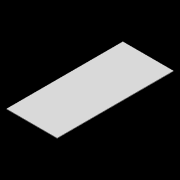
# Autodesk Inventor part: AirPlate
Saved by Autodesk Inventor 2022 (Build 260153000, 153)
## iProperties
Created: 2021-10-09
Part Number: AirPlate
Material: Generic
Document SubType Name: Modeling
Designer: timmy
Density: 1 g/cm^3
Appearance: Default
Author: timmy
Autodesk Inventor part; units mm, degrees
ref_plane "YZ Plane" through (0, 0, 0) normal (1, 0, 0) x (0, 1, 0)
ref_plane "XZ Plane" through (0, 0, 0) normal (0, 1, 0) x (-1, 0, 0)
ref_plane "XY Plane" through (0, 0, 0) normal (0, 0, 1) x (1, 0, 0)
sketch "Sketch1" plane through (0, 0, 0) normal (0, 1, 0) x (-1, 0, 0)
  line L0 (0, 0) -> (188.2648, 0)
  line L1 (188.2648, 0) -> (188.2648, -431.8)
  line L2 (188.2648, -431.8) -> (0, -431.8)
  line L3 (0, -431.8) -> (0, 0)
  dimension "d0" = 188.2648
  dimension "d1" = 431.8
  constraints: 8 end point, 2 parallel, 1 horizontal, 1 perpendicular
  measures "d0" distance of L1.end L2.end
  measures "d1" distance of L0.end L1.end
extrude "Extrusion1" add sketch "Sketch1" along normal blind 1.5875
body "Solid1"
